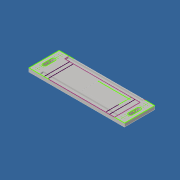
# Autodesk Inventor part: Button Fixture Base
Saved by Autodesk Inventor 2016 (Build 200138000, 138)
## iProperties
Created: 2016-07-07
Part Number: Button Fixture Base
Material: Generic
Document SubType Name: Modeling
Designer: Sam Clay
Density: 1 g/cm^3
Appearance: Default
Author: Sam Clay
Autodesk Inventor part; units mm, degrees
ref_plane "YZ Plane" through (0, 0, 0) normal (1, 0, 0) x (0, 1, 0)
ref_plane "XZ Plane" through (0, 0, 0) normal (0, 1, 0) x (-1, 0, 0)
ref_plane "XY Plane" through (0, 0, 0) normal (0, 0, 1) x (1, 0, 0)
sketch "Sketch1" plane through (0, 0, 0) normal (0, 1, 0) x (-1, 0, 0)
  line L0 (0, 0) -> (381, 0)
  line L1 (381, 0) -> (381, 152.4)
  line L2 (381, 152.4) -> (0, 152.4)
  line L3 (0, 152.4) -> (0, 0)
  line L4 (381, 0) -> (431.8, 0)
  line L5 (431.8, 0) -> (431.8, 152.4)
  line L6 (431.8, 152.4) -> (381, 152.4)
  line L7 (381, 152.4) -> (381, 0)
  line L8 (0, 0) -> (-50.8, 0)
  line L9 (-50.8, 0) -> (-50.8, 152.4)
  line L10 (-50.8, 152.4) -> (0, 152.4)
  line L11 (0, 152.4) -> (0, 0)
  dimension "d0" = 381
  dimension "d1" = 152.4
  dimension "d2" = 50.8
  dimension "d3" = 50.8
  constraints: 24 end point, 6 parallel, 3 horizontal, 3 perpendicular, 2 point on line
  measures "d0" distance of L2.end L1.end
  measures "d1" distance of L1.end L0.end
  measures "d2" distance of L6.end L5.end
  measures "d3" distance of L9.end L10.end
extrude "Extrusion1" add sketch "Sketch1" along normal blind 19.05 contours L3 L2 L1 L0
extrude "Extrusion2" add sketch "Sketch1" along normal blind 17.78 contours L8 L9 L10 L3 | L1 L6 L5 L4
sketch "Sketch2" plane through (0, 19.05, 0) normal (0, 1, 0) x (1, 0, 0)
  line L0 (-381, 0) -> (-381, -152.4) projected
  line L1 (0, 0) -> (-381, 0)
  line L2 (-381, 0) -> (-381, -3.175)
  line L3 (-381, -3.175) -> (0, -3.175)
  line L4 (0, -3.175) -> (0, 0)
  line L5 (0, -3.175) -> (-381, -3.175)
  line L6 (-381, -3.175) -> (-381, -22.987)
  line L7 (-381, -22.987) -> (0, -22.987)
  line L8 (0, -22.987) -> (0, -3.175)
  line L9 (0, -22.987) -> (-381, -22.987)
  line L10 (-381, -22.987) -> (-381, -35.687)
  line L11 (-381, -35.687) -> (0, -35.687)
  line L12 (0, -35.687) -> (0, -22.987)
  line L13 (0, -35.687) -> (-381, -35.687)
  line L14 (-381, -35.687) -> (-381, -116.967)
  line L15 (-381, -116.967) -> (0, -116.967)
  line L16 (0, -116.967) -> (0, -35.687)
  line L17 (0, -116.967) -> (-381, -116.967)
  line L18 (-381, -116.967) -> (-381, -129.667)
  line L19 (-381, -129.667) -> (0, -129.667)
  line L20 (0, -129.667) -> (0, -116.967)
  line L21 (0, -129.667) -> (-381, -129.667)
  line L22 (-381, -129.667) -> (-381, -149.479)
  line L23 (-381, -149.479) -> (0, -149.479)
  line L24 (0, -149.479) -> (0, -129.667)
  line L25 (0, -149.479) -> (-381, -149.479)
  line L26 (-381, -149.479) -> (-381, -152.654)
  line L27 (-381, -152.654) -> (0, -152.654)
  line L28 (0, -152.654) -> (0, -149.479)
  line L29 (0, -152.4) -> (0, 0) projected
  line L30 (0, 0) -> (-44.45, 0)
  line L31 (-44.45, 0) -> (-44.45, -116.967)
  line L32 (-44.45, -116.967) -> (0, -116.967)
  line L33 (0, -116.967) -> (0, 0)
  circle A0 centre (-48.1046, -38.862) radius 8.89
  line L34 (-44.45, -35.687) -> (-199.39, -35.687)
  line L35 (-199.39, -35.687) -> (-199.39, -116.967)
  line L36 (-199.39, -116.967) -> (-44.45, -116.967)
  line L37 (-44.45, -116.967) -> (-44.45, -35.687)
  dimension "d8" = 3.175
  dimension "d9" = 19.812
  dimension "d10" = 12.7
  dimension "d11" = 81.28
  dimension "d12" = 12.7
  dimension "d13" = 19.812
  dimension "d14" = 3.175
  dimension "d15" = 44.45
  dimension "d16" = 17.78
  dimension "d21" = 3.175
  dimension "d49" = 154.94
  constraints: 72 end point, 18 parallel, 11 point on line, 9 horizontal, 9 perpendicular, 1 centre point
  measures "d8" distance of L2.end L1.end
  measures "d9" distance of L6.end L5.end
  measures "d10" distance of L10.end L9.end
  measures "d11" distance of L14.end L13.end
  measures "d12" distance of L18.end L17.end
  measures "d13" distance of L22.end L21.end
  measures "d14" distance of L26.end L25.end
  measures "d15" distance of L32.end L31.end
  measures "d16" diameter of A0
  measures "d21" distance from line of L13 A0.centre
  measures "d49" distance of L36.end L35.end
extrude "Extrusion3" cut sketch "Sketch2" against normal blind 9.525 contours L3 L31 L7 L0 | L3 L8 L7 L31 | L19 L24 L23 L0
extrude "Extrusion4" cut sketch "Sketch2" against normal blind 1.5875 contours L11 A0 L31 L15 L35 | A0 L11 L31 | L31 L11 A0 | L11 L31 A0 | L11 A0 L31
sketch "Sketch3" plane through (0, 19.05, 0) normal (0, 1, 0) x (1, 0, 0)
  line L0 (50.8, -152.4) -> (50.8, 0)
  line L1 (50.8, 0) -> (0, 0)
  line L2 (0, -152.4) -> (50.8, -152.4)
  line L3 (-431.8, 0) -> (-431.8, -152.4)
  line L4 (-355.6, 0) -> (-431.8, 0)
  line L5 (-431.8, -152.4) -> (-330.2, -152.4)
  line L6 (-406.4, -54.102) -> (-406.4, -98.552) construction
  line L7 (-415.925, -54.102) -> (-415.925, -98.552)
  line L8 (-396.875, -98.552) -> (-396.875, -54.102)
  arc A0 (-396.875, -54.102) -> (-415.925, -54.102) centre (-406.4, -54.102) ccw
  arc A1 (-415.925, -98.552) -> (-396.875, -98.552) centre (-406.4, -98.552) ccw
  line L9 (25.4, -54.102) -> (25.4, -98.552) construction
  line L10 (15.875, -54.102) -> (15.875, -98.552)
  line L11 (34.925, -98.552) -> (34.925, -54.102)
  arc A2 (34.925, -54.102) -> (15.875, -54.102) centre (25.4, -54.102) ccw
  arc A3 (15.875, -98.552) -> (34.925, -98.552) centre (25.4, -98.552) ccw
  line L12 (-177.8, -35.687) -> (-37.282, -35.687)
  line L13 (-44.45, -27.3491) -> (-44.45, -98.586)
  line L14 (-431.8, -152.4) -> (-381, -152.4)
  line L15 (0, -152.4) -> (50.8, -152.4)
  line L16 (50.8, 0) -> (0, 0)
  line L17 (50.8, -152.4) -> (50.8, 0)
  line L18 (-431.8, 0) -> (-431.8, -152.4)
  line L19 (-199.39, -35.687) -> (-56.4083, -35.687)
  line L20 (-44.45, -46.9661) -> (-44.45, -116.967)
  point P0 (-44.45, -35.687)
  point P1 (25.4, -19.05)
  point P2 (25.4, -38.1)
  point P3 (25.4, -133.35)
  point P4 (25.4, -114.3)
  point P5 (-406.4, -19.05)
  point P6 (-406.4, -38.1)
  point P7 (-406.4, -133.35)
  point P8 (-406.4, -114.3)
  point P9 (-406.4, -76.327)
  point P10 (25.4, -76.327)
  dimension "d22" = 25.4
  dimension "d23" = 19.05
  dimension "d24" = 19.05
  dimension "d25" = 25.4
  dimension "d26" = 19.05
  dimension "d27" = 19.05
  dimension "d28" = 25.4
  dimension "d29" = 25.4
  dimension "d30" = 25.4
  dimension "d31" = 19.05
  dimension "d33" = 19.05
  dimension "d34" = 19.05
  dimension "d35" = 19.05
  dimension "d36" = 25.4
  dimension "d37" = 25.4
  dimension "d38" = 25.4
  dimension "d39" = 44.45
  dimension "d40" = 19.05
  dimension "d43" = 44.45
  dimension "d44" = 19.05
  dimension "d53" = 25.4
  constraints: 46 end point, 8 point on circle, 8 tangent, 7 collinear, 4 centre point, 2 midpoint, 2 parallel, 2 point on line, 2 vertical
  measures "d22" distance from line of L0 point (25.4, -19.05)
  measures "d23" distance from line of L1 point (25.4, -19.05)
  measures "d24" distance from line of L2 point (25.4, -133.35)
  measures "d25" distance from line of L0 point (25.4, -133.35)
  measures "d26" distance of point (25.4, -38.1) point (25.4, -19.05)
  measures "d27" distance of point (25.4, -114.3) point (25.4, -133.35)
  measures "d28" distance from line of L0 point (25.4, -114.3)
  measures "d29" distance from line of L0 point (25.4, -38.1)
  measures "d30" distance from line of L3 point (-406.4, -19.05)
  measures "d31" distance from line of L4 point (-406.4, -19.05)
  measures "d33" distance of point (-406.4, -19.05) point (-406.4, -38.1)
  measures "d34" distance of point (-406.4, -133.35) point (-406.4, -114.3)
  measures "d35" distance from line of L5 point (-406.4, -133.35)
  measures "d36" distance from line of L3 point (-406.4, -38.1)
  measures "d37" distance from line of L3 point (-406.4, -114.3)
  measures "d38" distance from line of L3 point (-406.4, -133.35)
  measures "d39" distance of L6.start L6.end
  measures "d40" diameter of A1
  measures "d43" distance of L9.start L9.end
  measures "d44" diameter of A3
  measures "d53" distance from line of point (-406.4, -76.327) L3
extrude "Extrusion5" cut sketch "Sketch3" against normal through all
sketch "Sketch4" plane through (0, 19.05, 0) normal (0, 1, 0) x (1, 0, 0)
  line L0 (0, -22.987) -> (-381, -22.987) projected
  line L1 (-355.6, -22.987) -> (-355.6, -152.4)
  line L2 (-25.4, -22.987) -> (-25.4, -152.4)
  line L3 (-381, -22.987) -> (-381, -3.175) projected
  line L4 (0, -152.4) -> (0, -22.987) projected
  line L5 (-336.55, -22.987) -> (-336.55, -152.4)
  line L6 (-381, -152.4) -> (0, -152.4) projected
  line L7 (-44.45, -22.987) -> (-44.45, -152.4)
  point P0 (0, 0)
  dimension "d50" = 25.4
  dimension "d51" = 25.4
  dimension "d52" = 19.05
  dimension "d55" = 19.05
  constraints: 8 end point, 8 point on line, 2 vertical, 1 parallel
  measures "d50" distance between parallel lines of L1 L3
  measures "d51" distance between parallel lines of L2 L4
  measures "d52" distance between parallel lines of L5 L1
  measures "d55" distance between parallel lines of L7 L2
equation "\"d12\" = d10"
equation "\"d24\" = d23"
equation "\"d25\" = d22"
equation "\"d26\" = d23"
equation "\"d27\" = d26"
equation "\"d28\" = d22"
equation "\"d29\" = d22"
equation "\"d30\" = d22"
equation "\"d31\" = d23"
equation "\"d33\" = d31"
equation "\"d34\" = d31"
equation "\"d35\" = d31"
equation "\"d36\" = d22"
equation "\"d37\" = d22"
equation "\"d38\" = d22"
equation "\"d39\" = d43"
equation "\"d40\" = d44"
body "Solid1"
